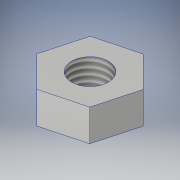
# Autodesk Inventor part: nut for sqrew long
Saved by Autodesk Inventor 2018 (Build 220112000, 112)
## iProperties
Created: 2018-03-02
Part Number: nut for sqrew long
Material: Aluminum 6061
Document SubType Name: Modeling
Designer: 238438
Density: 2.7 g/cm^3
Appearance: Aluminum - Flat
Mass: 0.0463623 g
Surface Area: 0.530531 cm^2
Volume: 0.0171712 cm^3
Author: 238438
Autodesk Inventor part; units mm, degrees
ref_plane "YZ Plane" through (0, 0, 0) normal (1, 0, 0) x (0, 1, 0)
ref_plane "XZ Plane" through (0, 0, 0) normal (0, 1, 0) x (-1, 0, 0)
ref_plane "XY Plane" through (0, 0, 0) normal (0, 0, 1) x (1, 0, 0)
sketch "Sketch1" plane through (0, 0, 0) normal (0, 1, 0) x (-1, 0, 0)
  line L0 (-1.5905, 1.6033) -> (0.5932, 2.1791)
  line L1 (0.5932, 2.1791) -> (2.1837, 0.5758)
  line L2 (2.1837, 0.5758) -> (1.5905, -1.6033)
  line L3 (1.5905, -1.6033) -> (-0.5932, -2.1791)
  line L4 (-0.5932, -2.1791) -> (-2.1837, -0.5758)
  line L5 (-2.1837, -0.5758) -> (-1.5905, 1.6033)
  circle A0 centre (0, 0) radius 0.9525
  dimension "d0" = 3.9116
  dimension "d1" = 1.905
  constraints: 12 end point, 2 coincident, 1 centre point, 13 other
  measures "d0" distance between parallel lines of L3 L0
  measures "d1" diameter of A0
extrude "Extrusion1" add sketch "Sketch1" along normal blind 1.651
thread "Thread1" size "0-80 UNF" class "2B" standard "ANSI Unified Screw Threads" full length
body "Solid1"
